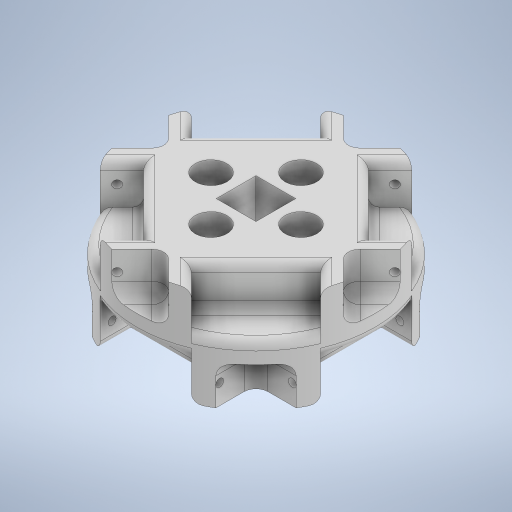
# Autodesk Inventor part: omni-wheel
Saved by Autodesk Inventor 2024.2 (Build 282272000, 272)
## iProperties
Created: 2024-04-01
Part Number: omni-wheel
Material: Generic
Document SubType Name: Modeling
Designer: Robin
Density: 1 g/cm^3
Appearance: Default
Author: Robin
Autodesk Inventor part; units mm, degrees
ref_plane "YZ Plane" through (0, 0, 0) normal (1, 0, 0) x (0, 1, 0)
ref_plane "XZ Plane" through (0, 0, 0) normal (0, 1, 0) x (-1, 0, 0)
ref_plane "XY Plane" through (0, 0, 0) normal (0, 0, 1) x (1, 0, 0)
sketch "Sketch1" plane through (0, 0, 0) normal (0, 1, 0) x (-1, 0, 0)
  circle A0 centre (0, 0) radius 30
  dimension "d0" = 60
  constraints: 1 centre point, 1 coincident
  measures "d0" diameter of A0
extrude "Extrusion1" add sketch "Sketch1" along normal blind 25
sketch "Sketch2" plane through (0, 25, 0) normal (0, 1, 0) x (1, 0, 0)
  line L0 (0, -16.2635) -> (-29.3449, 13.0815)
  line L1 (-29.3449, 13.0815) -> (-13.0815, 29.3449)
  line L2 (-13.0815, 29.3449) -> (0, 16.2635)
  line L3 (0, 16.2635) -> (0, -16.2635)
  line L4 (0, 0) -> (-21.2132, 21.2132)
  line L5 (-22.2739, 6.0104) -> (-6.0104, 22.2739)
  circle A0 centre (0, 0) radius 30 projected
  dimension "d3" = 23
  dimension "d5" = 45
  dimension "d6" = 10
  constraints: 12 end point, 3 perpendicular, 2 coincident, 2 midpoint, 2 point on line, 2 other
  measures "d3" distance of L0.end L1.end
  measures "d5" angle of L0 L3
  measures "d6" distance between parallel lines of L1 L5
extrude "Extrusion2" cut sketch "Sketch2" against normal blind 10 contours L0 A0 L4 L5 | L0 L1 A0 | L4 A0 L2 L5 | L1 L2 A0
sketch "Sketch3" plane through (0, 0, 0) normal (0, -1, 0) x (1, 0, 0)
  line L0 (30, 11.5) -> (0, 11.5)
  line L1 (0, 11.5) -> (0, -11.5)
  line L2 (0, -11.5) -> (30, -11.5)
  line L3 (30, -11.5) -> (30, 11.5)
  line L4 (20, 11.5) -> (20, -11.5)
  circle A0 centre (0, 0) radius 30 projected
  dimension "d12" = 23
  dimension "d14" = 10
  constraints: 10 end point, 2 coincident, 2 parallel, 2 perpendicular, 2 point on line, 1 horizontal, 1 midpoint, 1 tangent
  measures "d12" distance of L2.end L0.start
  measures "d14" distance between parallel lines of L3 L4
extrude "Extrusion3" cut sketch "Sketch3" against normal blind 10 contours L0 A0 L2 L4 | L0 L3 A0 | L3 L2 A0
sketch "Sketch4" plane through (20, 0, -11.5) normal (0, 0, 1) x (1, 0, 0)
  circle A0 centre (4.7083, 5) radius 1
  line L0 (7.7083, 0) -> (-50, 0) projected
  point P0 (-20, 0)
  dimension "d17" = 5
  dimension "d18" = 3
  dimension "d19" = 2
  constraints: 1 centre point
  measures "d17" distance from line of L0 A0.centre
  measures "d18" horizontal distance of L0.start A0.centre
  measures "d19" diameter of A0
extrude "Extrusion4" cut sketch "Sketch4" along normal through all both and the other way through all
fillet "Fillet1" radius 2 5 edges at (20, 0, 0) (23.8542, 0, -11.5) (23.8542, 0, 11.5) (20, 10, 0) (30, 10, 0)
pattern_circular "Circular Pattern2" count 4 over 360 about axis through (0, 0, 0) along (0, 1, 0) of "Extrusion3", "Fillet1", "Extrusion4"
sketch "Sketch5" plane through (-27.7245, 15, -11.461) normal (0.7071068, 0, -0.7071068) x (-0.7071068, 0, -0.7071068)
  circle A0 centre (-3, 5) radius 1
  line L0 (0, 10) -> (-57.7083, 10) projected
  line L1 (0, 10) -> (0, 0) projected
  point P0 (-27.7083, -15)
  dimension "d26" = 5
  dimension "d28" = 2
  dimension "d39" = 3
  constraints: 1 centre point
  measures "d26" distance from line of L0 A0.centre
  measures "d28" diameter of A0
  measures "d39" distance from line of L1 A0.centre
extrude "Extrusion5" cut sketch "Sketch5" along normal through all both and the other way through all
fillet "Fillet2" radius 2 5 edges at (-14.1421, 25, -14.1421) (-14.1421, 15, -14.1421) (-24.9992, 25, -8.7357) (-8.7357, 25, -24.9992) (-21.2132, 15, -21.2132)
pattern_circular "Circular Pattern3" count 4 over 360 about axis through (0, 0, 0) along (0, 1, 0) of "Fillet2", "Extrusion2", "Extrusion5"
sketch "Sketch6" plane through (0, 0, 0) normal (0, -1, 0) x (1, 0, 0)
  line L0 (5, 5) -> (-5, 5)
  line L1 (-5, 5) -> (-5, -5)
  line L2 (-5, -5) -> (5, -5)
  line L3 (5, -5) -> (5, 5)
  point P0 (0, 0)
  point P1 (5, 0)
  point P2 (0, -5)
  dimension "d35" = 10
  dimension "d36" = 10
  constraints: 8 end point, 2 midpoint, 2 parallel, 1 horizontal, 1 horizontal alignment, 1 perpendicular, 1 vertical alignment
  measures "d35" distance of L2.end L0.start
  measures "d36" distance of L1.end L2.end
extrude "Extrusion6" cut sketch "Sketch6" against normal through all
sketch "Sketch7" plane through (0, 25, 0) normal (0, 1, 0) x (1, 0, 0)
  line L0 (-14.1421, 36.1421) -> (0, 22)
  line L1 (-11.5, 22) -> (11.5, 22) projected
  line L2 (14.1421, 36.1421) -> (0, 22)
  line L3 (-14.1421, 36.1421) -> (14.1421, 36.1421)
  line L4 (-3.182, 22.2739) -> (-9.3981, 28.4899) projected
  point P0 (0, 0)
  dimension "d40" = 90
  dimension "d41" = 45
  dimension "d42" = 20
  constraints: 6 end point, 1 midpoint, 1 parallel
  measures "d40" angle of L2 L0
  measures "d41" angle of L3 L0
  measures "d42" distance of L0.start L0.end
extrude "Extrusion7" cut sketch "Sketch7" against normal blind 10
fillet "Fillet3" radius 3 3 edges at (0, 20, -22) (3.5692, 15, -25.5692) (-3.5692, 15, -25.5692)
pattern_circular "Circular Pattern4" count 4 over 360 about axis through (0, 0, 0) along (0, 1, 0) of "Extrusion7", "Fillet3"
sketch "Sketch8" plane through (0, 0, 0) normal (0, -1, 0) x (1, 0, 0)
  line L0 (-23.6881, 7.4246) -> (-7.4246, 23.6881) projected
  line L1 (-15.5563, 15.5563) -> (-35.5563, 15.5563)
  line L2 (-35.5563, 15.5563) -> (-35.5563, 35.5563)
  line L3 (-35.5563, 35.5563) -> (-15.5563, 35.5563)
  line L4 (-15.5563, 35.5563) -> (-15.5563, 15.5563)
  point P0 (0, 0)
  dimension "d49" = 20
  dimension "d50" = 20
  constraints: 8 end point, 2 parallel, 1 horizontal, 1 midpoint, 1 perpendicular
  measures "d49" distance of L2.end L3.end
  measures "d50" distance of L1.end L2.end
extrude "Extrusion8" cut sketch "Sketch8" against normal blind 10
fillet "Fillet4" radius 3 3 edges at (-20.6039, 10, 15.5563) (-15.5563, 5, 15.5563) (-15.5563, 10, 20.6039)
pattern_circular "Circular Pattern5" count 4 over 360 about axis through (0, 0, 0) along (0, 1, 0) of "Extrusion8", "Fillet4"
sketch "Sketch9" plane through (0, 25, 0) normal (0, 1, 0) x (1, 0, 0)
  circle A0 centre (11.3137, 0) radius 4
  line L0 (22.2739, -3.182) -> (3.182, -22.2739) projected
  line L1 (3.182, 22.2739) -> (22.2739, 3.182) projected
  point P0 (0, 0)
  dimension "d57" = 8
  dimension "d58" = 10
  dimension "d59" = 10
  constraints: 1 centre point
  measures "d57" diameter of A0
  measures "d58" distance from line of L0 A0.centre
  measures "d59" distance from line of L1 A0.centre
extrude "Extrusion9" cut sketch "Sketch9" against normal through all
pattern_circular "Circular Pattern6" count 4 over 360 about axis through (0, 0, 0) along (0, 1, 0) of "Extrusion9"
body "Solid1"
